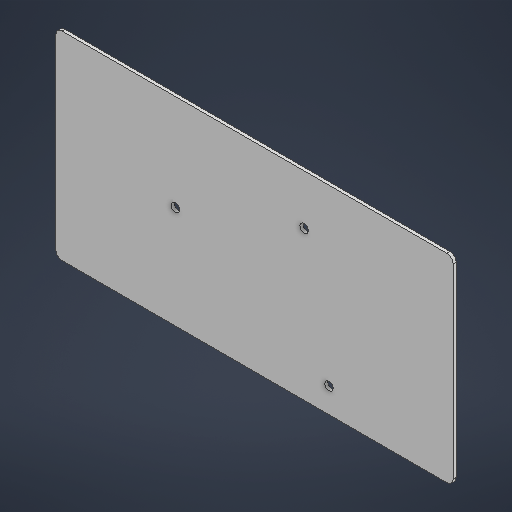
# Autodesk Inventor part: smalleraligner
Saved by Autodesk Inventor 2026.1 (Build 301233000, 233)
## iProperties
Created: 2026-03-30
Part Number: smalleraligner
Material: Generic
Document SubType Name: Modeling
Designer: roejo
Density: 1 g/cm^3
Appearance: Default
Author: roejo
Autodesk Inventor part; units mm, degrees
ref_plane "YZ Plane" through (0, 0, 0) normal (1, 0, 0) x (0, 1, 0)
ref_plane "XZ Plane" through (0, 0, 0) normal (0, 1, 0) x (-1, 0, 0)
ref_plane "XY Plane" through (0, 0, 0) normal (0, 0, 1) x (1, 0, 0)
sketch "Sketch1" plane through (0, 0, 0) normal (0, 0, 1) x (1, 0, 0)
  line L0 (99.3506, 56.5591) -> (-97.4994, 56.5591)
  line L1 (-100.6744, 53.3841) -> (-100.6744, -41.8659)
  line L2 (-97.4994, -45.0409) -> (99.3506, -45.0409)
  line L3 (102.5256, -41.8659) -> (102.5256, 53.3841)
  circle A0 centre (26.3256, 31.1591) radius 2.1844
  circle A1 centre (-39.484, 7.4002) radius 2.1844
  circle A2 centre (39.0256, -32.3409) radius 2.1844
  arc A3 (99.3506, -45.0409) -> (102.5256, -41.8659) centre (99.3506, -41.8659) ccw
  arc A4 (102.5256, 53.3841) -> (99.3506, 56.5591) centre (99.3506, 53.3841) ccw
  arc A5 (-97.4994, 56.5591) -> (-100.6744, 53.3841) centre (-97.4994, 53.3841) ccw
  arc A6 (-100.6744, -41.8659) -> (-97.4994, -45.0409) centre (-97.4994, -41.8659) ccw
  point P0 (0, 0)
  point P1 (-100.6744, -45.0409)
  point P2 (-100.6744, 56.5591)
  point P3 (102.5256, -45.0409)
  dimension "d0" = 203.2
  dimension "d1" = 101.6
  dimension "d2" = 25.4
  dimension "d3" = 76.2
  dimension "d4" = 3.175
  constraints: 8 end point, 8 point on circle, 8 tangent, 7 centre point, 6 point on line, 3 equal radius, 2 parallel, 1 horizontal, 1 perpendicular
  measures "d0" distance of point (102.526, -45.041) point (-100.674, -45.041)
  measures "d1" distance of point (-100.674, -45.041) point (-100.674, 56.559)
  measures "d2" distance from line of L0 A0.centre
  measures "d3" distance from line of L3 A0.centre
  measures "d4" radius of A3
extrude "Extrusion1" add sketch "Sketch1" along normal blind 1.5875
body "Solid1"
